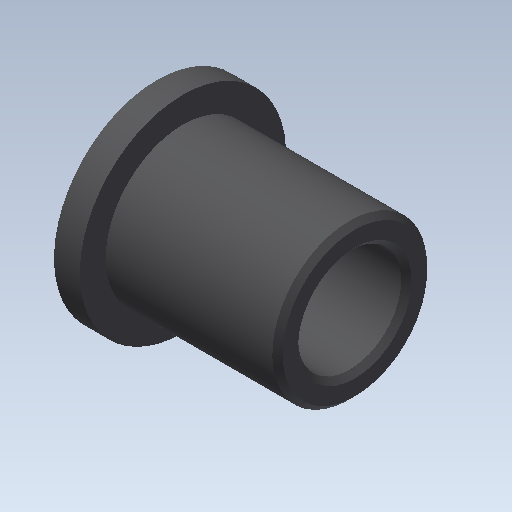
# Autodesk Inventor part: TFZF6-10
Saved by Autodesk Inventor 2020 (Build 240168000, 168)
## iProperties
Created: 2017-02-10
Part Number: TFZF6-10
Catalog Web Link: www.cadenas.de
Description: TFZF-Oil Free Bushings - PTFE - Flanged
Vendor: MISUMI
Document SubType Name: Modeling
Designer: psAdmin
Manufacturer: MISUMI
Mass: 0.477667 g
Surface Area: 7.14231 cm^2
Volume: 0.477667 cm^3
Density: 1 g/cm^3
Material: Generic
Appearance: PSOLRGB-175-175-175
Category: PARTsolutions
Company: MISUMI
PSOL_IDENT_0: {$CADENAS_DATA\23d-libs\misumi\metric\05_oil_free_bushings\tfzf.prj},148 {VTYP=3D},{NB=TFZF6-10},{LI
PSOL_IDENT_1: NA=TFZF6-10},{NN=TFZF},{DATE=17.06.2016 05:45:44},{GEOMDATE=13.02.2014},{VERSION=},{LINEID=90},{LINE
PSOL_IDENT_2: SUBID=-1},{WBVAR=L}  {NB=TFZF6-10},{LINA=TFZF6-10},{KT=DUMMY},{PN=TFZF6-10},{MAT=PTFE},{TR=-200~200}
PSOL_IDENT_3: ,{DD=6},{DDTOL=+0.182/+0.132},{L=10},{LTOL=0/-0.25},{L1=5,8,10},{D=9},{DTOL=+0.090/+0.040},{HS=9},{H
PSOL_IDENT_4: STOL=+0.015/0},{TOL=+0.125/+0.075},{SIZE=6},{SIZETOL=-0.004/-0.012},{F=12},{T=1.5},{AA=C0.3},{C=0.3}
NN: TFZF
NT: Oil Free Bushings - PTFE - Flanged
NB: TFZF6-10
NBSYN: $PN.
LINA: TFZF6-10
PN: TFZF6-10
MAT: PTFE
TR: -200~200
DD: 6
DDTOL: +0.182/+0.132
L: 10
LTOL: 0/-0.25
D: 9
DTOL: +0.090/+0.040
HS: 9
HSTOL: +0.015/0
TOL: +0.125/+0.075
SIZE: 6
SIZETOL: -0.004/-0.012
F: 12
T: 1.5
AA: C0.3
SUPPLIER: MISUMI
ARTICLENO: TFZF6-10
BOMINFO: TFZF6-10
CREATOR: CADENAS GmbH
Title: TFZF6-10
Author: Cadenas PARTsolutions
Comments: Oil Free Bushings - PTFE - Flanged
Autodesk Inventor part; units mm, degrees
ref_plane "YZ Plane" through (0, 0, 0) normal (1, 0, 0) x (0, 1, 0)
ref_plane "XZ Plane" through (0, 0, 0) normal (0, 1, 0) x (-1, 0, 0)
ref_plane "XY Plane" through (0, 0, 0) normal (0, 0, 1) x (1, 0, 0)
sketch "Sketch_1" plane through (0, 0, 0) normal (0, 0, 1) x (1, 0, 0)
  line L0 (11.5, 0) -> (0, 0)
  line L1 (0, 6) -> (0, 3.3)
  line L2 (0, 3.3) -> (0.3, 3)
  line L3 (0.3, 3) -> (11.2, 3)
  line L4 (11.2, 3) -> (11.5, 3.3)
  line L5 (11.5, 3.3) -> (11.5, 4.2)
  line L6 (11.5, 4.2) -> (11.2, 4.5)
  line L7 (11.2, 4.5) -> (1.5, 4.5)
  line L8 (1.5, 4.5) -> (1.5, 6)
  line L9 (1.5, 6) -> (0, 6)
  constraints: 20 end point
revolve "Revolution1" add sketch "Sketch_1" angle 360 about axis through (11.5, 0, 0) along (1, 0, 0)
body "Solid1"
